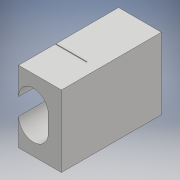
# Autodesk Inventor part: Cutting Tool V1
Saved by Autodesk Inventor 2017 (Build 210142000, 142)
## iProperties
Created: 2018-11-11
Part Number: Cutting Tool V1
Material: Generic
Document SubType Name: Modeling
Designer: djenl
Density: 1 g/cm^3
Appearance: Default
Author: djenl
Autodesk Inventor part; units mm, degrees
ref_plane "YZ Plane" through (0, 0, 0) normal (1, 0, 0) x (0, 1, 0)
ref_plane "XZ Plane" through (0, 0, 0) normal (0, 1, 0) x (-1, 0, 0)
ref_plane "XY Plane" through (0, 0, 0) normal (0, 0, 1) x (1, 0, 0)
sketch "Sketch1" plane through (0, 0, 0) normal (0, 0, 1) x (1, 0, 0)
  line L0 (-7.5, 17.5) -> (7.5, 17.5)
  line L1 (7.5, 17.5) -> (7.5, -17.5)
  line L2 (7.5, -17.5) -> (-7.5, -17.5)
  line L3 (-7.5, -17.5) -> (-7.5, 17.5)
  line L4 (-7.5, 17.5) -> (7.5, -17.5) construction
  line L5 (7.5, 17.5) -> (-7.5, -17.5) construction
  point P0 (0, 0)
  dimension "d0" = 15
  dimension "d1" = 35
  constraints: 12 end point, 2 midpoint, 2 parallel, 1 horizontal, 1 perpendicular
  measures "d0" distance of L1.end L2.end
  measures "d1" distance of L0.end L1.end
extrude "Extrusion1" add sketch "Sketch1" along normal blind 25
sketch "Sketch2" plane through (-7.5, 17.5, 0) normal (0, 1, 0) x (1, 0, 0)
  line L0 (15, -25) -> (0, -25) construction
  line L1 (0, 0) -> (10.4, 0) construction
  line L2 (10.4, 0) -> (10.4, -25) construction
  line L3 (10.4, -25) -> (0, -25) construction
  line L4 (0, -25) -> (0, 0) construction
  line L5 (0, 0) -> (15, 0) construction
  line L6 (5.2, 0) -> (5.2, -25) construction
  line L7 (10.4, -12.5) -> (0, -12.5) construction
  line L8 (0, 0) -> (0, -25) construction
  line L9 (10.4, -4.3) -> (0, -4.3) construction
  line L10 (0, -4.3) -> (0, -20.7) construction
  line L11 (0, -20.7) -> (10.4, -20.7) construction
  line L12 (10.4, -20.7) -> (10.4, -4.3) construction
  line L13 (10.4, -4.3) -> (0, -20.7) construction
  line L14 (0, -4.3) -> (10.4, -20.7) construction
  circle A0 centre (5.2, -9.5) radius 5.2
  circle A1 centre (5.2, -15.5) radius 5.2
  line L15 (10.4, -9.5) -> (0, -9.5)
  line L16 (0, -9.5) -> (0, -15.5)
  line L17 (0, -15.5) -> (10.4, -15.5)
  line L18 (10.4, -15.5) -> (10.4, -9.5)
  line L19 (10.4, -9.5) -> (0, -15.5) construction
  line L20 (0, -9.5) -> (10.4, -15.5) construction
  point P0 (7.5, 0)
  point P1 (5.2, -12.5)
  dimension "d4" = 10.4
  dimension "d5" = 16.4
  constraints: 36 end point, 8 midpoint, 6 parallel, 4 horizontal, 4 point on line, 3 perpendicular, 3 tangent, 2 vertical, 1 centre point, 1 horizontal alignment, 2 other
  measures "d4" distance of L2.end L3.end
  measures "d5" distance of L10.end L9.end
extrude "Extrusion2" cut sketch "Sketch2" against normal blind 35
sketch "Sketch3" plane through (-7.5, -17.5, 0) normal (-1, 0, 0) x (0, 0, 1)
  line L0 (25, 35) -> (25, 0) projected
  line L1 (0, 0) -> (0, 35) projected
  line L2 (25, 13.0367) -> (0, 13.0367)
  line L3 (0, 13.0367) -> (0, 12.8367)
  line L4 (0, 12.8367) -> (25, 12.8367)
  line L5 (25, 12.8367) -> (25, 13.0367)
  point P0 (0, 17.5)
  dimension "d8" = 0.2
  constraints: 8 end point, 2 parallel, 2 point on line, 1 horizontal, 1 perpendicular
  measures "d8" distance of L3.end L2.end
extrude "Extrusion3" cut sketch "Sketch3" against normal blind 11
body "Solid1"
